Autodesk Inventor part; units mm, degrees
(part 2 of 2)
  arc A460 (-11.5976, -8.718) -> (-11.9305, -8.668) centre (-11.7894, -8.8622) ccw
  line L233 (-11.9305, -8.668) -> (-13.9623, -10.1442)
  arc A461 (-11.6207, -9.0791) -> (-11.577, -8.7453) centre (-11.7685, -8.89) ccw
  arc A462 (-11.5976, -8.718) -> (-11.577, -8.7453) centre (0, 0) ccw
  line L234 (0, 0) -> (-14.5082, -9.7859) construction
  line L235 (-14.3078, -9.6507) -> (-12.2184, -8.2414)
  arc A463 (-13.5998, -10.6253) -> (-13.639, -10.9648) centre (-13.452, -10.8144) ccw
  arc A464 (-13.639, -10.9648) -> (-13.5609, -11.0613) centre (0, 0) ccw
  arc A465 (-13.5609, -11.0613) -> (-13.2206, -11.0934) centre (-13.3749, -10.9096) ccw
  arc A466 (-10.9612, -9.5057) -> (-11.2968, -9.4791) centre (-11.1425, -9.663) ccw
  line L236 (-11.2968, -9.4791) -> (-13.2206, -11.0934)
  arc A467 (-10.9591, -9.8676) -> (-10.9387, -9.5316) centre (-11.1197, -9.6892) ccw
  arc A468 (-10.9612, -9.5057) -> (-10.9387, -9.5316) centre (0, 0) ccw
  line L237 (0, 0) -> (-13.7902, -10.7741) construction
  line L238 (-13.5998, -10.6253) -> (-11.6137, -9.0736)
  arc A469 (-12.8254, -11.5481) -> (-12.841, -11.8895) centre (-12.6648, -11.7264) ccw
  arc A470 (-12.841, -11.8895) -> (-12.7563, -11.9803) centre (0, 0) ccw
  arc A471 (-12.7563, -11.9803) -> (-12.4146, -11.9886) centre (-12.5813, -11.816) ccw
  arc A472 (-10.2714, -10.2472) -> (-10.608, -10.244) centre (-10.4413, -10.4167) ccw
  line L239 (-10.608, -10.244) -> (-12.4146, -11.9886)
  arc A473 (-10.244, -10.608) -> (-10.2472, -10.2714) centre (-10.4167, -10.4413) ccw
  arc A474 (-10.2714, -10.2472) -> (-10.2472, -10.2714) centre (0, 0) ccw
  line L240 (0, 0) -> (-13.005, -11.7098) construction
  line L241 (-12.8254, -11.5481) -> (-10.9525, -9.8617)
  arc A475 (-11.9886, -12.4146) -> (-11.9803, -12.7563) centre (-11.816, -12.5813) ccw
  arc A476 (-11.9803, -12.7563) -> (-11.8895, -12.841) centre (0, 0) ccw
  arc A477 (-11.8895, -12.841) -> (-11.5481, -12.8254) centre (-11.7264, -12.6648) ccw
  arc A478 (-9.5316, -10.9387) -> (-9.8676, -10.9591) centre (-9.6892, -11.1197) ccw
  line L242 (-9.8676, -10.9591) -> (-11.5481, -12.8254)
  arc A479 (-9.4791, -11.2968) -> (-9.5057, -10.9612) centre (-9.663, -11.1425) ccw
  arc A480 (-9.5316, -10.9387) -> (-9.5057, -10.9612) centre (0, 0) ccw
  line L243 (0, 0) -> (-12.1565, -12.5884) construction
  line L244 (-11.9886, -12.4146) -> (-10.2379, -10.6017)
  arc A481 (-11.0934, -13.2206) -> (-11.0613, -13.5609) centre (-10.9096, -13.3749) ccw
  arc A482 (-11.0613, -13.5609) -> (-10.9648, -13.639) centre (0, 0) ccw
  arc A483 (-10.9648, -13.639) -> (-10.6253, -13.5998) centre (-10.8144, -13.452) ccw
  arc A484 (-8.7453, -11.577) -> (-9.0791, -11.6207) centre (-8.89, -11.7685) ccw
  line L245 (-9.0791, -11.6207) -> (-10.6253, -13.5998)
  arc A485 (-8.668, -11.9305) -> (-8.718, -11.5976) centre (-8.8622, -11.7894) ccw
  arc A486 (-8.7453, -11.577) -> (-8.718, -11.5976) centre (0, 0) ccw
  line L246 (0, 0) -> (-11.2488, -13.4058) construction
  line L247 (-11.0934, -13.2206) -> (-9.4734, -11.29)
  arc A487 (-10.1442, -13.9623) -> (-10.0884, -14.2995) centre (-9.95, -14.1034) ccw
  arc A488 (-10.0884, -14.2995) -> (-9.9867, -14.3707) centre (0, 0) ccw
  arc A489 (-9.9867, -14.3707) -> (-9.6507, -14.3078) centre (-9.8497, -14.1736) ccw
  arc A490 (-7.9164, -12.1588) -> (-8.2464, -12.2257) centre (-8.0474, -12.3599) ccw
  line L248 (-8.2464, -12.2257) -> (-9.6507, -14.3078)
  arc A491 (-7.8147, -12.5061) -> (-7.8877, -12.1775) centre (-8.0182, -12.3789) ccw
  arc A492 (-7.9164, -12.1588) -> (-7.8877, -12.1775) centre (0, 0) ccw
  line L249 (0, 0) -> (-10.2862, -14.1578) construction
  line L250 (-10.1442, -13.9623) -> (-8.6628, -11.9233)
  arc A493 (-9.1455, -14.6359) -> (-9.0663, -14.9684) centre (-8.942, -14.7631) ccw
  arc A494 (-9.0663, -14.9684) -> (-8.9599, -15.0323) centre (0, 0) ccw
  arc A495 (-8.9599, -15.0323) -> (-8.6292, -14.9462) centre (-8.837, -14.8262) ccw
  arc A496 (-7.049, -12.6814) -> (-7.3734, -12.7712) centre (-7.1656, -12.8912) ccw
  line L251 (-7.3734, -12.7712) -> (-8.6292, -14.9462)
  arc A497 (-6.9232, -13.0207) -> (-7.019, -12.698) centre (-7.1352, -12.9081) ccw
  arc A498 (-7.049, -12.6814) -> (-7.019, -12.698) centre (0, 0) ccw
  line L252 (0, 0) -> (-9.2736, -14.8408) construction
  line L253 (-9.1455, -14.6359) -> (-7.81, -12.4986)
  arc A499 (-8.1023, -15.2382) -> (-8.0001, -15.5643) centre (-7.8904, -15.3509) ccw
  arc A500 (-8.0001, -15.5643) -> (-7.8895, -15.6207) centre (0, 0) ccw
  arc A501 (-7.8895, -15.6207) -> (-7.5656, -15.5117) centre (-7.7813, -15.4065) ccw
  arc A502 (-6.1472, -13.1422) -> (-6.4646, -13.2544) centre (-6.2489, -13.3596) ccw
  line L254 (-6.4646, -13.2544) -> (-7.5656, -15.5117)
  arc A503 (-5.9981, -13.472) -> (-6.1162, -13.1567) centre (-6.2173, -13.3743) ccw
  arc A504 (-6.1472, -13.1422) -> (-6.1162, -13.1567) centre (0, 0) ccw
  line L255 (0, 0) -> (-8.2158, -15.4516) construction
  line L256 (-8.1023, -15.2382) -> (-6.9191, -13.0129)
  arc A505 (-7.0196, -15.7663) -> (-6.8949, -16.0845) centre (-6.8003, -15.8639) ccw
  arc A506 (-6.8949, -16.0845) -> (-6.7806, -16.133) centre (0, 0) ccw
  arc A507 (-6.7806, -16.133) -> (-6.4651, -16.0016) centre (-6.6876, -15.9117) ccw
  arc A508 (-5.2155, -13.539) -> (-5.5243, -13.6731) centre (-5.3018, -13.763) ccw
  line L257 (-5.5243, -13.6731) -> (-6.4651, -16.0016)
  arc A509 (-5.0437, -13.8575) -> (-5.1835, -13.5513) centre (-5.2693, -13.7755) ccw
  arc A510 (-5.2155, -13.539) -> (-5.1835, -13.5513) centre (0, 0) ccw
  line L258 (0, 0) -> (-7.1179, -15.987) construction
  line L259 (-7.0196, -15.7663) -> (-5.9945, -13.4639)
  arc A511 (-5.9027, -16.2175) -> (-5.7561, -16.5263) centre (-5.6772, -16.2996) ccw
  arc A512 (-5.7561, -16.5263) -> (-5.6387, -16.5667) centre (0, 0) ccw
  arc A513 (-5.6387, -16.5667) -> (-5.3331, -16.4136) centre (-5.5614, -16.3395) ccw
  arc A514 (-4.2583, -13.8699) -> (-4.557, -14.0251) centre (-4.3288, -14.0993) ccw
  line L260 (-4.557, -14.0251) -> (-5.3331, -16.4136)
  arc A515 (-4.0648, -14.1756) -> (-4.2256, -13.8799) centre (-4.2955, -14.1095) ccw
  arc A516 (-4.2583, -13.8699) -> (-4.2256, -13.8799) centre (0, 0) ccw
  line L261 (0, 0) -> (-5.9854, -16.4446) construction
  line L262 (-5.9027, -16.2175) -> (-5.0407, -13.8492)
  arc A517 (-4.757, -16.5898) -> (-4.5893, -16.8875) centre (-4.5263, -16.6559) ccw
  arc A518 (-4.5893, -16.8875) -> (-4.4693, -16.9197) centre (0, 0) ccw
  arc A519 (-4.4693, -16.9197) -> (-4.1752, -16.7457) centre (-4.408, -16.6876) ccw
  arc A520 (-3.2805, -14.1331) -> (-3.5676, -14.3088) centre (-3.3347, -14.3669) ccw
  line L263 (-3.5676, -14.3088) -> (-4.1752, -16.7457)
  arc A521 (-3.066, -14.4246) -> (-3.2471, -14.1408) centre (-3.3008, -14.3747) ccw
  arc A522 (-3.2805, -14.1331) -> (-3.2471, -14.1408) centre (0, 0) ccw
  line L264 (0, 0) -> (-4.8237, -16.8221) construction
  line L265 (-4.757, -16.5898) -> (-4.0624, -14.1671)
  arc A523 (-3.5882, -16.8812) -> (-3.4001, -17.1665) centre (-3.3535, -16.9311) ccw
  arc A524 (-3.4001, -17.1665) -> (-3.2782, -17.1902) centre (0, 0) ccw
  arc A525 (-3.2782, -17.1902) -> (-2.9969, -16.9961) centre (-3.2332, -16.9545) ccw
  arc A526 (-2.2866, -14.3275) -> (-2.5608, -14.5228) centre (-2.3244, -14.5645) ccw
  line L266 (-2.5608, -14.5228) -> (-2.9969, -16.9961)
  arc A527 (-2.0524, -14.6034) -> (-2.2528, -14.3329) centre (-2.29, -14.57) ccw
  arc A528 (-2.2866, -14.3275) -> (-2.2528, -14.3329) centre (0, 0) ccw
  line L267 (0, 0) -> (-3.6385, -17.1176) construction
  line L268 (-3.5882, -16.8812) -> (-3.0642, -14.416)
  arc A529 (-2.4019, -17.0904) -> (-2.1943, -17.3619) centre (-2.1642, -17.1238) ccw
  arc A530 (-2.1943, -17.3619) -> (-2.0711, -17.377) centre (0, 0) ccw
  arc A531 (-2.0711, -17.377) -> (-1.804, -17.1638) centre (-2.0427, -17.1387) ccw
  arc A532 (-1.2816, -14.4521) -> (-1.5415, -14.6661) centre (-1.3028, -14.6912) ccw
  line L269 (-1.5415, -14.6661) -> (-1.804, -17.1638)
  arc A533 (-1.0287, -14.711) -> (-1.2475, -14.4551) centre (-1.2681, -14.6942) ccw
  arc A534 (-1.2816, -14.4521) -> (-1.2475, -14.4551) centre (0, 0) ccw
  line L270 (0, 0) -> (-2.4355, -17.3297) construction
  line L271 (-2.4019, -17.0904) -> (-2.0511, -14.5946)
  arc A535 (-1.2039, -17.2163) -> (-0.9779, -17.4727) centre (-0.9645, -17.233) ccw
  arc A536 (-0.9779, -17.4727) -> (-0.8539, -17.4792) centre (0, 0) ccw
  arc A537 (-0.8539, -17.4792) -> (-0.6023, -17.2478) centre (-0.8422, -17.2394) ccw
  arc A538 (-0.2703, -14.5063) -> (-0.5147, -14.7379) centre (-0.2748, -14.7463) ccw
  line L272 (-0.5147, -14.7379) -> (-0.6023, -17.2478)
  arc A539 (0, -14.7469) -> (-0.2361, -14.5069) centre (-0.24, -14.7469) ccw
  arc A540 (-0.2703, -14.5063) -> (-0.2361, -14.5069) centre (0, 0) ccw
  line L273 (0, 0) -> (-1.2207, -17.4574) construction
  line L274 (-1.2039, -17.2163) -> (-1.0281, -14.7021)
  arc A541 (0.2433, -17.4983) -> (0.3675, -17.4961) centre (0, 0) ccw
  arc A542 (1.4634, -17.4387) -> (1.5871, -17.4279) centre (0, 0) ccw
  arc A543 (2.6763, -17.2941) -> (2.7989, -17.2747) centre (0, 0) ccw
  arc A544 (3.8761, -17.0653) -> (3.9971, -17.0374) centre (0, 0) ccw
  arc A545 (5.0571, -16.7534) -> (5.1758, -16.7171) centre (0, 0) ccw
  arc A546 (6.2134, -16.3598) -> (6.3294, -16.3153) centre (0, 0) ccw
  arc A547 (7.3395, -15.8865) -> (7.452, -15.834) centre (0, 0) ccw
  arc A548 (8.4298, -15.3358) -> (8.5384, -15.2756) centre (0, 0) ccw
  arc A549 (9.4791, -14.7105) -> (9.5832, -14.6428) centre (0, 0) ccw
  arc A550 (10.4821, -14.0134) -> (10.5813, -13.9387) centre (0, 0) ccw
  arc A551 (11.4341, -13.2481) -> (11.5278, -13.1666) centre (0, 0) ccw
  arc A552 (12.3304, -12.4182) -> (12.4182, -12.3304) centre (0, 0) ccw
  arc A553 (13.1666, -11.5278) -> (13.2481, -11.4341) centre (0, 0) ccw
  arc A554 (13.9387, -10.5813) -> (14.0134, -10.4821) centre (0, 0) ccw
  arc A555 (14.6428, -9.5832) -> (14.7105, -9.4791) centre (0, 0) ccw
  arc A556 (15.2756, -8.5384) -> (15.3358, -8.4298) centre (0, 0) ccw
  arc A557 (15.834, -7.452) -> (15.8865, -7.3395) centre (0, 0) ccw
  arc A558 (16.3153, -6.3294) -> (16.3598, -6.2134) centre (0, 0) ccw
  arc A559 (16.7171, -5.1758) -> (16.7534, -5.0571) centre (0, 0) ccw
  arc A560 (17.0374, -3.9971) -> (17.0653, -3.8761) centre (0, 0) ccw
  arc A561 (17.2747, -2.7989) -> (17.2941, -2.6763) centre (0, 0) ccw
  arc A562 (17.4279, -1.5871) -> (17.4387, -1.4634) centre (0, 0) ccw
  arc A563 (17.4961, -0.3675) -> (17.4983, -0.2433) centre (0, 0) ccw
  arc A564 (17.4792, 0.8539) -> (17.4727, 0.9779) centre (0, 0) ccw
  arc A565 (17.377, 2.0711) -> (17.3619, 2.1943) centre (0, 0) ccw
  arc A566 (17.1902, 3.2782) -> (17.1665, 3.4001) centre (0, 0) ccw
  arc A567 (16.9197, 4.4693) -> (16.8875, 4.5893) centre (0, 0) ccw
  arc A568 (16.5667, 5.6387) -> (16.5263, 5.7561) centre (0, 0) ccw
  arc A569 (16.133, 6.7806) -> (16.0845, 6.8949) centre (0, 0) ccw
  arc A570 (15.6207, 7.8895) -> (15.5643, 8.0001) centre (0, 0) ccw
  arc A571 (15.0323, 8.9599) -> (14.9684, 9.0663) centre (0, 0) ccw
  arc A572 (14.3707, 9.9867) -> (14.2995, 10.0884) centre (0, 0) ccw
  arc A573 (13.639, 10.9648) -> (13.5609, 11.0613) centre (0, 0) ccw
  arc A574 (12.841, 11.8895) -> (12.7563, 11.9803) centre (0, 0) ccw
  arc A575 (11.9803, 12.7563) -> (11.8895, 12.841) centre (0, 0) ccw
  arc A576 (11.0613, 13.5609) -> (10.9648, 13.639) centre (0, 0) ccw
  arc A577 (10.0884, 14.2995) -> (9.9867, 14.3707) centre (0, 0) ccw
  arc A578 (9.0663, 14.9684) -> (8.9599, 15.0323) centre (0, 0) ccw
  arc A579 (8.0001, 15.5643) -> (7.8895, 15.6207) centre (0, 0) ccw
  arc A580 (6.8949, 16.0845) -> (6.7806, 16.133) centre (0, 0) ccw
  arc A581 (5.7561, 16.5263) -> (5.6387, 16.5667) centre (0, 0) ccw
  arc A582 (4.5893, 16.8875) -> (4.4693, 16.9197) centre (0, 0) ccw
  arc A583 (3.4001, 17.1665) -> (3.2782, 17.1902) centre (0, 0) ccw
  arc A584 (2.1943, 17.3619) -> (2.0711, 17.377) centre (0, 0) ccw
  arc A585 (0.9779, 17.4727) -> (0.8539, 17.4792) centre (0, 0) ccw
  arc A586 (-0.2433, 17.4983) -> (-0.3675, 17.4961) centre (0, 0) ccw
  arc A587 (-1.4634, 17.4387) -> (-1.5871, 17.4279) centre (0, 0) ccw
  arc A588 (-2.6763, 17.2941) -> (-2.7989, 17.2747) centre (0, 0) ccw
  arc A589 (-3.8761, 17.0653) -> (-3.9971, 17.0374) centre (0, 0) ccw
  arc A590 (-5.0571, 16.7534) -> (-5.1758, 16.7171) centre (0, 0) ccw
  arc A591 (-6.2134, 16.3598) -> (-6.3294, 16.3153) centre (0, 0) ccw
  arc A592 (-7.3395, 15.8865) -> (-7.452, 15.834) centre (0, 0) ccw
  arc A593 (-8.4298, 15.3358) -> (-8.5384, 15.2756) centre (0, 0) ccw
  arc A594 (-9.4791, 14.7105) -> (-9.5832, 14.6428) centre (0, 0) ccw
  arc A595 (-10.4821, 14.0134) -> (-10.5813, 13.9387) centre (0, 0) ccw
  arc A596 (-11.4341, 13.2481) -> (-11.5278, 13.1666) centre (0, 0) ccw
  arc A597 (-12.3304, 12.4182) -> (-12.4182, 12.3304) centre (0, 0) ccw
  arc A598 (-13.1666, 11.5278) -> (-13.2481, 11.4341) centre (0, 0) ccw
  arc A599 (-13.9387, 10.5813) -> (-14.0134, 10.4821) centre (0, 0) ccw
  arc A600 (-14.6428, 9.5832) -> (-14.7105, 9.4791) centre (0, 0) ccw
  arc A601 (-15.2756, 8.5384) -> (-15.3358, 8.4298) centre (0, 0) ccw
  arc A602 (-15.834, 7.452) -> (-15.8865, 7.3395) centre (0, 0) ccw
  arc A603 (-16.3153, 6.3294) -> (-16.3598, 6.2134) centre (0, 0) ccw
  arc A604 (-16.7171, 5.1758) -> (-16.7534, 5.0571) centre (0, 0) ccw
  arc A605 (-17.0374, 3.9971) -> (-17.0653, 3.8761) centre (0, 0) ccw
  arc A606 (-17.2747, 2.7989) -> (-17.2941, 2.6763) centre (0, 0) ccw
  arc A607 (-17.4279, 1.5871) -> (-17.4387, 1.4634) centre (0, 0) ccw
  arc A608 (-17.4961, 0.3675) -> (-17.4983, 0.2433) centre (0, 0) ccw
  arc A609 (-17.4792, -0.8539) -> (-17.4727, -0.9779) centre (0, 0) ccw
  arc A610 (-17.377, -2.0711) -> (-17.3619, -2.1943) centre (0, 0) ccw
  arc A611 (-17.1902, -3.2782) -> (-17.1665, -3.4001) centre (0, 0) ccw
  arc A612 (-16.9197, -4.4693) -> (-16.8875, -4.5893) centre (0, 0) ccw
  arc A613 (-16.5667, -5.6387) -> (-16.5263, -5.7561) centre (0, 0) ccw
  arc A614 (-16.133, -6.7806) -> (-16.0845, -6.8949) centre (0, 0) ccw
  arc A615 (-15.6207, -7.8895) -> (-15.5643, -8.0001) centre (0, 0) ccw
  arc A616 (-15.0323, -8.9599) -> (-14.9684, -9.0663) centre (0, 0) ccw
  arc A617 (-14.3707, -9.9867) -> (-14.2995, -10.0884) centre (0, 0) ccw
  arc A618 (-13.639, -10.9648) -> (-13.5609, -11.0613) centre (0, 0) ccw
  arc A619 (-12.841, -11.8895) -> (-12.7563, -11.9803) centre (0, 0) ccw
  arc A620 (-11.9803, -12.7563) -> (-11.8895, -12.841) centre (0, 0) ccw
  arc A621 (-11.0613, -13.5609) -> (-10.9648, -13.639) centre (0, 0) ccw
  arc A622 (-10.0884, -14.2995) -> (-9.9867, -14.3707) centre (0, 0) ccw
  arc A623 (-9.0663, -14.9684) -> (-8.9599, -15.0323) centre (0, 0) ccw
  arc A624 (-8.0001, -15.5643) -> (-7.8895, -15.6207) centre (0, 0) ccw
  arc A625 (-6.8949, -16.0845) -> (-6.7806, -16.133) centre (0, 0) ccw
  arc A626 (-5.7561, -16.5263) -> (-5.6387, -16.5667) centre (0, 0) ccw
  arc A627 (-4.5893, -16.8875) -> (-4.4693, -16.9197) centre (0, 0) ccw
  arc A628 (-3.4001, -17.1665) -> (-3.2782, -17.1902) centre (0, 0) ccw
  arc A629 (-2.1943, -17.3619) -> (-2.0711, -17.377) centre (0, 0) ccw
  arc A630 (-0.9779, -17.4727) -> (-0.8539, -17.4792) centre (0, 0) ccw
  point P0 (17.5, 0)
  point P1 (17.5, 0)
  point P2 (17.2941, -2.6763)
  point P3 (17.4279, -1.5871)
  point P4 (14.6661, -1.5415)
  point P5 (17.0653, -3.8761)
  point P6 (17.2747, -2.7989)
  point P7 (14.5228, -2.5608)
  point P8 (16.7534, -5.0571)
  point P9 (17.0374, -3.9971)
  point P10 (14.3088, -3.5676)
  point P11 (16.3598, -6.2134)
  point P12 (16.7171, -5.1758)
  point P13 (14.0251, -4.557)
  point P14 (15.8865, -7.3395)
  point P15 (16.3153, -6.3294)
  point P16 (13.6731, -5.5243)
  point P17 (15.3358, -8.4298)
  point P18 (15.834, -7.452)
  point P19 (14.7105, -9.4791)
  point P20 (15.2756, -8.5384)
  point P21 (12.7712, -7.3734)
  point P22 (14.0134, -10.4821)
  point P23 (14.6428, -9.5832)
  point P24 (12.2257, -8.2464)
  point P25 (13.2481, -11.4341)
  point P26 (13.9387, -10.5813)
  point P27 (12.4182, -12.3304)
  point P28 (13.1666, -11.5278)
  point P29 (10.9591, -9.8676)
  point P30 (11.5278, -13.1666)
  point P31 (12.3304, -12.4182)
  point P32 (10.5813, -13.9387)
  point P33 (9.4791, -11.2968)
  point P34 (9.5832, -14.6428)
  point P35 (10.4821, -14.0134)
  point P36 (8.668, -11.9305)
  point P37 (8.5384, -15.2756)
  point P38 (9.4791, -14.7105)
  point P39 (7.8147, -12.5061)
  point P40 (7.452, -15.834)
  point P41 (8.4298, -15.3358)
  point P42 (6.9232, -13.0207)
  point P43 (6.3294, -16.3153)
  point P44 (7.3395, -15.8865)
  point P45 (5.9981, -13.472)
  point P46 (5.1758, -16.7171)
  point P47 (3.9971, -17.0374)
  point P48 (2.7989, -17.2747)
  point P49 (3.066, -14.4246)
  point P50 (1.5871, -17.4279)
  point P51 (2.6763, -17.2941)
  point P52 (2.0524, -14.6034)
  point P53 (0.3675, -17.4961)
  point P54 (-0.8539, -17.4792)
  point P55 (0.2433, -17.4983)
  point P56 (0, -14.7469)
  point P57 (-2.0711, -17.377)
  point P58 (-0.9779, -17.4727)
  point P59 (-3.2782, -17.1902)
  point P60 (-2.1943, -17.3619)
  point P61 (-2.0524, -14.6034)
  point P62 (-4.4693, -16.9197)
  point P63 (-3.4001, -17.1665)
  point P64 (-3.066, -14.4246)
  point P65 (-5.6387, -16.5667)
  point P66 (-4.5893, -16.8875)
  point P67 (-6.7806, -16.133)
  point P68 (-5.7561, -16.5263)
  point P69 (-5.0437, -13.8575)
  point P70 (-7.8895, -15.6207)
  point P71 (-6.8949, -16.0845)
  point P72 (-5.9981, -13.472)
  point P73 (-8.9599, -15.0323)
  point P74 (-8.0001, -15.5643)
  point P75 (-9.9867, -14.3707)
  point P76 (-9.0663, -14.9684)
  point P77 (-7.8147, -12.5061)
  point P78 (-10.9648, -13.639)
  point P79 (-10.0884, -14.2995)
  point P80 (-8.668, -11.9305)
  point P81 (-12.7563, -11.9803)
  point P82 (-11.9803, -12.7563)
  point P83 (-11.8895, -12.841)
  point P84 (-11.0613, -13.5609)
  point P85 (-17.3619, -2.1943)
  point P86 (-17.1902, -3.2782)
  point P87 (-17.1665, -3.4001)
  point P88 (-16.9197, -4.4693)
  point P89 (-16.8875, -4.5893)
  point P90 (-16.5667, -5.6387)
  point P91 (-16.5263, -5.7561)
  point P92 (-16.133, -6.7806)
  point P93 (-13.6731, -5.5243)
  point P94 (-16.0845, -6.8949)
  point P95 (-15.6207, -7.8895)
  point P96 (-15.5643, -8.0001)
  point P97 (-15.0323, -8.9599)
  point P98 (-12.7712, -7.3734)
  point P99 (-14.9684, -9.0663)
  point P100 (-14.3707, -9.9867)
  point P101 (-14.2995, -10.0884)
  point P102 (-13.639, -10.9648)
  point P103 (-13.5609, -11.0613)
  point P104 (-12.841, -11.8895)
  dimension "d24" = 0.5
  dimension "d25" = 2
  dimension "d26" = 2
  dimension "d27" = 2
  dimension "d29" = 0.24
  dimension "d32" = 360
  dimension "d36" = 360
  constraints: 1352 point on circle, 630 centre point, 550 end point, 93 coincident, 93 point on line, 7 tangent, 1 collinear, 1 vertical, 2613 other
  measures "d24" distance of L4.end L2.end
  measures "d25" angle of L1 L2
  measures "d26" angle of L4 L3
  measures "d27" angle of L7 L6
  measures "d29" radius of A6
extrude "Extrusion3" cut sketch "Skizze5" against normal through all contours A0 A123 L65 A124 A126 A125 L70 A127 | A0 A117 L62 A118 A120 A119 L67 A121 | A0 A111 L59 A112 A114 A113 L64 A115 | A0 A105 L56 A106 A108 A107 L61 A109 | A0 A99 L53 A100 A102 A101 L58 A103 | A0 A93 L50 A94 A96 A95 L55 A97 | A0 A87 L47 A88 A90 A89 L52 A91 | A0 A81 L44 A82 A84 A83 L49 A85 | A0 A75 L41 A76 A78 A77 L46 A79 | A0 A69 L38 A70 A72 A71 L43 A73 | A0 A63 L35 A64 A66 A65 L40 A67 | A0 A57 L32 A58 A60 A59 L37 A61 | A0 A51 L29 A52 A54 A53 L34 A55 | A0 A45 L26 A46 A48 A47 L31 A49 | A0 A39 L23 A40 A42 A41 L28 A43 | A0 A33 L20 A34 A36 A35 L25 A37 | A0 A27 L17 A28 A30 A29 L22 A31 | A0 A21 L14 A22 A24 A23 L19 A25 | A0 A15 L11 A16 A18 A17 L16 A19 | A0 A9 L8 A10 A12 A11 L13 A13 | A0 A4 L5 A5 A2 A6 L10 A7 | A0 A537 L272 A538 A540 A539 L0 A3 | A0 A531 L269 A532 A534 A533 L274 A535 | A0 A525 L266 A526 A528 A527 L271 A529 | A0 A519 L263 A520 A522 A521 L268 A523 | A0 A513 L260 A514 A516 A515 L265 A517 | A0 A507 L257 A508 A510 A509 L262 A511 | A0 A501 L254 A502 A504 A503 L259 A505 | A0 A495 L251 A496 A498 A497 L256 A499 | A0 A489 L248 A490 A492 A491 L253 A493 | A0 A483 L245 A484 A486 A485 L250 A487 | A0 A477 L242 A478 A480 A479 L247 A481 | A0 A471 L239 A472 A474 A473 L244 A475 | A0 A465 L236 A466 A468 A467 L241 A469 | A0 A459 L233 A460 A462 A461 L238 A463 | A0 A453 L230 A454 A456 A455 L235 A457 | A0 A447 L227 A448 A450 A449 L232 A451 | A0 A441 L224 A442 A444 A443 L229 A445 | A0 A435 L221 A436 A438 A437 L226 A439 | A0 A429 L218 A430 A432 A431 L223 A433 | A0 A423 L215 A424 A426 A425 L220 A427 | A0 A417 L212 A418 A420 A419 L217 A421
pattern_circular "Runde Anordnung2" count 2 over 360 about axis through (0, 0, 0) along (0, 0, -1) of "Extrusion3"
